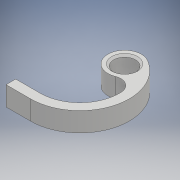
# Autodesk Inventor part: tablet_arm_joint
Saved by Autodesk Inventor 2018.3 (Build 223284000, 284)
## iProperties
Created: 2020-10-27
Part Number: tablet_arm_joint
Material: Generic
Document SubType Name: Modeling
Designer: chris
Density: 1 g/cm^3
Appearance: Default
Author: chris
Autodesk Inventor part; units mm, degrees
ref_plane "YZ Plane" through (0, 0, 0) normal (1, 0, 0) x (0, 1, 0)
ref_plane "XZ Plane" through (0, 0, 0) normal (0, 1, 0) x (-1, 0, 0)
ref_plane "XY Plane" through (0, 0, 0) normal (0, 0, 1) x (1, 0, 0)
sketch "Sketch1" plane through (0, 0, 0) normal (0, 0, 1) x (1, 0, 0)
  line L0 (0, -10) -> (25.4, -10)
  line L1 (25.4, 0) -> (0, 0)
  line L2 (0, 0) -> (0, -10)
  circle A0 centre (42.7, 70) radius 11.3
  arc A1 (51.5714, 84.8522) -> (49.2048, 53.9695) centre (42.7, 70) ccw
  arc A2 (25.4, -10) -> (51.5714, 84.8522) centre (25.4, 41.0367) ccw
  arc A3 (66.3907, 42.9781) -> (49.2048, 53.9695) centre (53.9047, 42.3867) ccw
  arc A4 (25.4, 0) -> (66.3907, 42.9781) centre (25.4, 41.0367) ccw
  point P0 (0, 0)
  point P1 (12.7, -10)
  point P2 (12.7, 0)
  constraints: 8 point on circle, 6 end point, 5 centre point, 2 horizontal, 2 midpoint, 2 tangent, 1 parallel, 5 other
extrude "Extrusion1" add sketch "Sketch1" along normal blind 20
chamfer "Chamfer2" distance 2 angle 45 2 edges at (31.4, 70, 20) (31.4, 70, 0)
body "Solid1"
